difonabase (Autodesk Fusion 360 design; units mm, degrees)
Autodesk Fusion 360 part; units mm, degrees
sketch "Sketch1" plane through (0, 0, 0) normal (0, 0, 1) x (1, 0, 0)
  circle A0 centre (0, 0) radius 35
  line L0 (0, 0) -> (0, 35)
  line L1 (0, 0) -> (-30.3109, -17.5)
  line L2 (0, 0) -> (30.3109, -17.5)
  circle A1 through (-29.7061, -20.0664, -4.307) (-32.8359, -13.1266, 0) (-28.3907, -19.307, 4.307)
  line L3 (-30.3109, -17.5) -> (-32.8109, -13.1699)
  line L4 (-30.3109, -17.5) -> (-25.3109, -17.5) construction
  circle A2 through (27.7859, -21.8734, 0) (30.9157, -14.9336, 4.307) (32.2311, -15.693, -4.307)
  circle A3 through (5.05, 35, 0) (-2.525, 34.2406, 4.307) (-2.525, 35.7594, -4.307)
  circle A4 centre (0, 0) radius 3
  dimension "d1" = 70
  dimension "d12" = 10.1
  dimension "d13" = 120
  dimension "d20" = 360
  dimension "d27" = 6
  constraint coincident A0.centre L0.start
  constraint coincident A0 L0.end
  constraint vertical L0
  constraint coincident L1.end L3.start
  constraint concentric A0 A4
  measures "d1" diameter of A0
  measures "d13" angle of L3 L4
  measures "d27" diameter of A4
sketch "Sketch3" plane through (0, 0, 0) normal (0, 1, 0) x (1, 0, 0)
  line L0 (-30.3109, 0) -> (-30.3109, 11.2222)
  line L1 (-30.3109, 11.2222) -> (-25, 12)
  line L2 (-25, 12) -> (0, 12)
  line L3 (0, 12) -> (0, 0)
  line L4 (-30.3109, 0) -> (-30.3109, -5.2495)
  line L5 (-30.3109, -5.2495) -> (0, -5.2495)
  line L6 (0, -5.2495) -> (0, 0)
  line L7 (-35, 0) -> (35, 0)
  point P0 (-30.3109, 0)
  dimension "d25" = 25
  dimension "d26" = 12
  constraint coincident P0 L0.start
  constraint vertical L0
  constraint perpendicular L0 L2
  constraint coincident L3.end L6.end
  constraint perpendicular L2 L3
  constraint parallel L0 L4
  constraint perpendicular L4 L5
  constraint perpendicular L5 L6
  measures "d25" distance of L1.end L2.end
  measures "d26" distance of L2 L7
revolve "Revolve1" add sketch "Sketch3" angle 360 about axis through (0, 0, 5.2495) along (0, 0, -1)
extrude "Extrude3" cut sketch "Sketch1" along normal blind 28 contours A1 in plane through (-29.3969, -16.9723, 5.9854) normal (0.852869, 0.492404, -0.173648)
extrude "Extrude4" cut sketch "Sketch1" against normal blind 28 contours A3 in plane through (0, 33.9446, 5.9854) normal (0, 0.984808, 0.173648)
extrude "Extrude5" cut sketch "Sketch1" against normal blind 28 contours A2 in plane through (29.3969, -16.9723, 5.9854) normal (0.852869, -0.492404, 0.173648)
extrude "Extrude6" cut sketch "Sketch1" along normal mid plane 30 contours L0 L2 A4 | L0 L1 A4 | L1 L2 A4
fillet "Fillet1" radius 1.2 2 edges at (-28.2597, 10.9609, -11.2222) (-28.2597, 10.9609, 5.2495)
